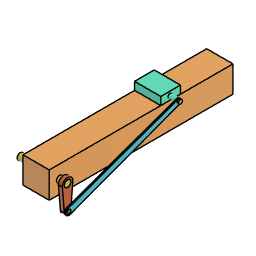
slider_crank (Autodesk Fusion 360 design; units mm, degrees)
part number: 2025-07-03-17-04-46-906
part number: 2025-07-03-17-09-40-898
part number: 2025-07-03-17-10-31-117
part number: 2025-07-03-17-13-40-289
part number: 2025-07-03-17-16-06-952
part number: 2025-07-03-17-55-16-241
Autodesk Fusion 360 part; units mm, degrees
sketch "Sketch1" plane through (0, 0, 0) normal (0, 1, 0) x (1, 0, 0)
  line L0 (15, -10) -> (115, -10)
  line L1 (115, -10) -> (115, -110)
  line L2 (115, -110) -> (15, -110)
  line L3 (15, -110) -> (15, -10)
  dimension "d1" = 100
  dimension "d2" = 100
  constraint horizontal L0
  constraint vertical L1
  constraint horizontal L2
  constraint vertical L3
  measures "d1" distance of L0.start L0.end
  measures "d2" distance of L0.start L2.end
extrude "Extrude1" add sketch "Sketch1" against normal blind 500 makes body 1 in component "Component"
sketch "Sketch2" plane through (0, 0, 0) normal (0, 1, 0) x (1, 0, 0)
  line L0 (115, -110) -> (15, -110)
  line L1 (15, -110) -> (15, -140)
  line L2 (15, -140) -> (115, -140)
  line L3 (115, -140) -> (115, -110)
  dimension "d5" = 30
  constraint horizontal L0
  constraint vertical L1
  constraint horizontal L2
  constraint vertical L3
  measures "d5" distance of L0.start L2.end
extrude "Extrude1'" add sketch "Sketch2" against normal blind 75 separate body makes body 2 in component "Component'"
sketch "Sketch3" plane through (115, 0, 0) normal (1, 0, 0) x (0, 1, 0)
  line L0 (0, 10) -> (0, 110)
  line L1 (0, 110) -> (-500, 110)
  line L2 (-500, 110) -> (-500, 10)
  line L3 (-500, 10) -> (0, 10)
  circle A0 centre (-460, 60) radius 12.5
  dimension "d8" = 25
  dimension "d9" = 50
  dimension "d10" = 40
  measures "d8" diameter of A0
  measures "d9" distance of L1 A0.centre
  measures "d10" distance of L2 A0.centre
extrude "Extrude2" cut sketch "Sketch3" against normal blind 200 contours A0 bodies 1 in component "Component"
extrude "Extrude1''" add sketch "Sketch3" along normal blind 30 and the other way blind 150 separate body contours A0 makes body 3 in component "Component''"
sketch "Sketch4" plane through (145, 0, 0) normal (1, 0, 0) x (0, 1, 0)
  circle A0 centre (-460, 60) radius 12.5
  circle A1 centre (-460, 60) radius 20
  circle A2 centre (-460, -30) radius 12.5
  line L0 (-479.9304, 58.3333) -> (-472.4565, -31.0417)
  line L1 (-440.0696, 58.3333) -> (-447.5435, -31.0417)
  circle A3 centre (-460, -30) radius 7.5
  dimension "d17" = 40
  dimension "d18" = 25
  dimension "d19" = 15
  dimension "d20" = 90
  constraint concentric A0 A1
  constraint coincident A1 L0.start
  constraint coincident A2 L0.end
  constraint tangent A2 L0
  constraint coincident A1 L1.start
  constraint coincident A2 L1.end
  constraint tangent A2 L1
  constraint tangent A1 L0
  constraint tangent A1 L1
  constraint concentric A2 A3
  measures "d17" diameter of A1
  measures "d18" diameter of A2
  measures "d19" diameter of A3
  measures "d20" distance of A0.centre A2.centre
extrude "Extrude1'''" add sketch "Sketch4" against normal blind 15 separate body makes body 4 in component "Component'''"
sketch "Sketch5" plane through (115, 0, 0) normal (1, 0, 0) x (0, 1, 0)
  line L0 (0, 110) -> (0, 140)
  line L1 (0, 140) -> (-75, 140)
  line L2 (-75, 140) -> (-75, 110)
  line L3 (-75, 110) -> (0, 110)
  circle A0 centre (-40, 125) radius 7.5
  dimension "d23" = 15
  dimension "d24" = 15
  dimension "d25" = 35
  measures "d23" diameter of A0
  measures "d24" distance of L1 A0.centre
  measures "d25" distance of L2 A0.centre
extrude "Extrude2'" add sketch "Sketch5" along normal blind 40 contours A0 bodies 2 in component "Component'"
sketch "Sketch6" plane through (115, 0, 0) normal (1, 0, 0) x (0, 1, 0)
  circle A0 centre (-40, 125) radius 7.5
sketch "Sketch7" plane through (115, 0, 0) normal (1, 0, 0) x (0, 1, 0)
sketch "Sketch8" plane through (155, 0, 0) normal (1, 0, 0) x (0, 1, 0)
  circle A0 centre (-40, 125) radius 7.5
sketch "Sketch9" plane through (145, 0, 0) normal (1, 0, 0) x (0, 1, 0)
  circle A0 centre (-460, 60) radius 12.5
  circle A1 centre (-460, -30) radius 7.5
  line L0 (-479.9304, 58.3333) -> (-472.4565, -31.0417)
  arc A2 (-472.4565, -31.0417) -> (-447.5435, -31.0417) centre (-460, -30) ccw
  line L1 (-447.5435, -31.0417) -> (-440.0696, 58.3333)
  arc A3 (-440.0696, 58.3333) -> (-479.9304, 58.3333) centre (-460, 60) ccw
  circle A4 centre (-460, -30) radius 12.5
  circle A5 centre (-41.2993, 123.3246) radius 10
  line L2 (-455.636, -41.7135) -> (-35, 115)
  line L3 (-464.2324, -18.2383) -> (-44.6852, 132.734)
  dimension "d34" = 25
  dimension "d35" = 20
  constraint concentric A1 A4
  constraint coincident A4 L2.start
  constraint coincident A2 L2.start
  constraint coincident A4 L3.start
  constraint coincident A5 L3.end
  constraint tangent A5 L3
  constraint tangent A5 L2
  constraint tangent A4 L3
  constraint tangent A4 L2
  measures "d34" diameter of A4
  measures "d35" diameter of A5
extrude "Extrude1''''" add sketch "Sketch9" along normal blind 5 separate body contours A2 A4 | A2 L1 A4 A5 L2 L3 | L1 A4 L3 | A5 makes body 5 in component "Component''''"
sketch "Sketch10" plane through (150, 0, 0) normal (1, 0, 0) x (0, 1, 0)
  arc A0 (-464.2324, -18.2383) -> (-455.636, -41.7135) centre (-460, -30) ccw
  line L0 (-455.636, -41.7135) -> (-37.8082, 113.9538)
  arc A1 (-37.8082, 113.9538) -> (-44.6852, 132.734) centre (-41.2993, 123.3246) ccw
  line L1 (-44.6852, 132.734) -> (-464.2324, -18.2383)
sketch "Sketch11" plane through (130, 0, 0) normal (-1, 0, 0) x (0, -1, 0)
  circle A0 centre (460, 60) radius 12.5
  circle A1 centre (460, -30) radius 7.5
  line L0 (472.4565, -31.0417) -> (479.9304, 58.3333)
  arc A2 (479.9304, 58.3333) -> (440.0696, 58.3333) centre (460, 60) ccw
  line L1 (440.0696, 58.3333) -> (447.5435, -31.0417)
  arc A3 (447.5435, -31.0417) -> (472.4565, -31.0417) centre (460, -30) ccw
  circle A4 through (459.5145, -37.4843, 0) (466.7228, -26.6782, 0.1409) (453.7627, -25.8375, -0.1409)
sketch "Sketch12" plane through (130, 0, 0) normal (-1, 0, 0) x (0, -1, 0)
extrude "Extrude2''" add sketch "Sketch11" against normal blind 20 contours A1 bodies 4 in component "Component'''"
sketch "Sketch13" plane through (130, 0, 0) normal (-1, 0, 0) x (0, -1, 0)
  circle A0 centre (460, 60) radius 12.5
  line L0 (472.4565, -31.0417) -> (479.9304, 58.3333)
  arc A1 (479.9304, 58.3333) -> (440.0696, 58.3333) centre (460, 60) ccw
  line L1 (440.0696, 58.3333) -> (447.5435, -31.0417)
  arc A2 (447.5435, -31.0417) -> (472.4565, -31.0417) centre (460, -30) ccw
  circle A3 centre (460, -30) radius 7.5
  dimension "d40" = 15
  constraint concentric A2 A3
  measures "d40" diameter of A3
extrude "Extrude3" cut sketch "Sketch13" against normal blind 5 contours A3 bodies 4 in component "Component'''"
move_body "Move1" bodies 5 to x (0.996195, 0, 0.087156) y (0, 1, 0) z (-0.087156, 0, 0.996195) at (9.8303, 0, -12.6691) in component "Component''''"
sketch "Sketch14" plane through (155.5632, 1.6953, 42.6527) normal (0.996195, 0, 0.087156) x (0, 1, 0)
  circle A0 centre (-461.6953, -72.4098) radius 7.5
  arc A1 (-465.9277, -60.6481) -> (-457.3313, -84.1233) centre (-461.6953, -72.4098) ccw
  line L0 (-457.3313, -84.1233) -> (-39.5035, 71.544)
  arc A2 (-39.5035, 71.544) -> (-46.3805, 90.3242) centre (-42.9946, 80.9148) ccw
  line L1 (-46.3805, 90.3242) -> (-465.9277, -60.6481)
extrude "Extrude2'''" cut sketch "Sketch8" against normal blind 25 bodies 5 in component "Component''''"
extrude "Extrude3'" add 1 faces at (48.3333, 0, 43.3333) along direction (0, 1, 0) blind 200 on bodies 1 bodies 1 in component "Component"
component "Component'" placed x (1, 0, 0) y (0, 1, 0) z (0, 0, 1) at (0, 0.0111, 0)
component "Component''" placed x (1, 0, 0) y (0, 1, 0) z (0, 0, 1) at (0, 0, 0)
component "Component'''" placed x (1, 0, 0) y (0, 1, -0.000171) z (0, 0.000171, 1) at (0, -0.0102, -0.0785)
component "Component''''" placed x (0.996195, -0.000015, -0.087156) y (0, 1, -0.000171) z (0.087156, 0.00017, 0.996195) at (-8.6887, -0.0079, 13.3992)
component "Component" placed x (1, 0, 0) y (0, 1, 0) z (0, 0, 1) at (0, 0, 0)
